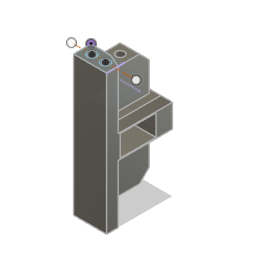
hinge_hood_front_v3 (Autodesk Fusion 360 design; units mm, degrees)
Autodesk Fusion 360 part; units mm, degrees
note: some values were not read from the file. Set by a fixed rule: which sketch regions a step uses.
sketch "Esquisse1" plane through (0, 0, 0) normal (0, 0, 1) x (1, 0, 0)
  line L0 (17, 0) -> (0, 0)
  line L1 (0, 0) -> (0, 72)
  line L2 (0, 72) -> (17, 72)
  line L3 (17, 72) -> (17, 0)
  dimension "d3" = 72
  dimension "d4" = 17
  constraint coincident L0.end L1.start
  constraint horizontal L0
  constraint perpendicular L0 L1
  constraint perpendicular L1 L2
  constraint perpendicular L0 L3
  measures "d3" distance of L0.end L1.end
  measures "d4" distance of L0.start L0.end
extrude "Extrusion1" add sketch "Esquisse1" along normal blind 9
sketch "Esquisse2" plane through (0, 0, 0) normal (0, -1, 0) x (1, 0, 0)
  line L0 (0, 0) -> (17, 0)
  line L1 (17, 9) -> (0, 9)
  line L2 (0, 9) -> (0, 0)
  line L3 (-5.7525, 4.5) -> (21.5406, 4.5) construction
  circle A0 centre (5, 4.5) radius 2.175
  circle A1 centre (12, 4.5) radius 2.175
  line L4 (17, 0) -> (17, 9)
  dimension "d7" = 4.35
  dimension "d8" = 7
  dimension "d9" = 4.5
  dimension "d10" = 5
  constraint coincident L3 A0.centre
  constraint coincident L3 A1.centre
  constraint equal A0 A1
  measures "d7" diameter of A0
  measures "d8" distance of A0.centre A1.centre
  measures "d9" vertical distance of L0.start L3.start
  measures "d10" distance of L2 A0.centre
extrude "Extrusion2" cut sketch "Esquisse2" against normal blind 8 contours A0 | A1
sketch "Esquisse3" plane through (0, 72, 0) normal (0, 1, 0) x (-1, 0, 0)
  line L0 (-17, 0) -> (0, 0)
  line L1 (0, 0) -> (0, 9)
  line L2 (0, 9) -> (-17, 9)
  line L3 (5.6122, 4.5) -> (-27.7174, 4.5) construction
  circle A0 centre (-12, 4.5) radius 2.175
  circle A1 centre (-5, 4.5) radius 2.175
  line L4 (-17, 9) -> (-17, 0)
  dimension "d13" = 4.5
  dimension "d14" = 7
  dimension "d15" = 5
  dimension "d16" = 4.35
  constraint coincident L3 A0.centre
  constraint coincident L3 A1.centre
  constraint equal A0 A1
  measures "d13" distance of L0.end L3
  measures "d14" distance of A0.centre A1.centre
  measures "d15" distance of L1 A1.centre
  measures "d16" diameter of A0
extrude "Extrusion3" cut sketch "Esquisse3" against normal blind 8 contours A0 | A1
sketch "Esquisse9" plane through (0, 0, 0) normal (-1, 0, 0) x (0, 0, 1)
  line L0 (0, 72) -> (0, 0)
  line L1 (0, 0) -> (9, 0)
  line L2 (9, 0) -> (9, 72)
  line L3 (9, 72) -> (0, 72)
  line L4 (9, 65) -> (-15, 65)
  line L5 (-15, 65) -> (-15, 48.5)
  line L6 (-15, 48.5) -> (9, 48.5)
  line L7 (9, 48.5) -> (9, 65)
  line L8 (9, 7) -> (-15, 7)
  line L9 (-15, 7) -> (-15, 23.5)
  line L10 (-15, 23.5) -> (9, 23.5)
  line L11 (9, 23.5) -> (9, 7)
  line L12 (6.675, 72) -> (2.325, 72)
  dimension "d48" = 7
  dimension "d49" = 7
  dimension "d50" = 25
  dimension "d51" = 15
  constraint horizontal L4
  constraint vertical L5
  constraint horizontal L6
  constraint vertical L7
  constraint coincident L2 L4.start
  constraint horizontal L8
  constraint vertical L9
  constraint horizontal L10
  constraint vertical L11
  constraint coincident L2 L8.start
  constraint equal L5 L9
  constraint collinear L5 L9
  measures "d48" distance of L1 L8
  measures "d49" distance of L4 L12
  measures "d50" distance of L6 L10
  measures "d51" distance of L0 L9
extrude "Extrusion7" add sketch "Esquisse9" against normal blind 10 contours L0 L4 L5 L6 | L0 L8 L9 L10
sketch "Esquisse10" plane through (0, 7, 0) normal (0, -1, 0) x (1, 0, 0)
  line L0 (0, -15) -> (10, -15)
  line L1 (10, -15) -> (10, 0)
  line L2 (10, 0) -> (0, 0)
  line L3 (0, 0) -> (0, -15)
  circle A0 centre (5, -10) radius 2.175
  dimension "d56" = 4.35
  dimension "d57" = 5
  dimension "d76" = 5
  measures "d56" diameter of A0
  measures "d57" distance of L0 A0.centre
  measures "d76" distance of L1 A0.centre
extrude "Extrusion9" cut sketch "Esquisse10" against normal blind 61 contours A0
sketch "Esquisse11" plane through (0, 48.5, 0) normal (0, -1, 0) x (1, 0, 0)
  circle A0 centre (5, -10) radius 2.175
  line L0 (10, -15) -> (10, 0)
  line L1 (10, 0) -> (0, 0)
  line L2 (0, 0) -> (0, -15)
  line L3 (0, -15) -> (10, -15)
chamfer "Chanfrein4" distance 7 distance2 3 1 edges at (17, 36, 0) measured on face at (3.3333, 40.1667, 0)
sketch "Esquisse12" plane through (0, 0, -15) normal (0, 0, -1) x (-1, 0, 0)
  line L0 (0, 48.5) -> (0, 65)
  line L1 (0, 65) -> (-10, 65)
  line L2 (-10, 65) -> (-10, 48.5)
  line L3 (-10, 48.5) -> (0, 48.5)
  line L4 (-10, 65) -> (0, 65)
  line L5 (0, 65) -> (0, 7)
  line L6 (0, 7) -> (-10, 7)
  line L7 (-10, 7) -> (-10, 65)
  line L8 (0, 7) -> (-10, 7)
  constraint horizontal L4
  constraint vertical L5
  constraint horizontal L6
  constraint vertical L7
  constraint coincident L1.end L2.start
  constraint collinear L6 L8
extrude "Extrusion10" add sketch "Esquisse12" along normal blind 10
extrude "Extrusion11" add 1 faces at (6.6667, 31.8333, -15) along direction (0, 0, 1) up to surface (15 mm away)
sketch "Esquisse13" plane through (0, 0, -25) normal (0, 0, -1) x (-1, 0, 0)
  line L0 (0, 7) -> (0, 65)
  line L1 (-10, 65) -> (-10, 7)
  line L2 (-10, 27) -> (-17, 27)
  line L3 (-17, 27) -> (-17, 45)
  line L4 (-17, 45) -> (-10, 45)
  line L5 (-10, 45) -> (-10, 27)
  line L6 (0, 65) -> (-10, 65)
  line L7 (-10, 7) -> (0, 7)
  dimension "d82" = 7
  constraint horizontal L2
  constraint vertical L3
  constraint horizontal L4
  constraint vertical L5
  constraint coincident L1 L2.start
  measures "d82" distance of L2.start L2.end
extrude "Extrusion12" add sketch "Esquisse13" against normal blind 28 contours L1 L2 L3 L4 L5
sketch "Esquisse15" plane through (17, 0, 0) normal (1, 0, 0) x (0, 0, -1)
  line L0 (-3, 45) -> (-3, 72)
  line L1 (-3, 72) -> (-9, 72)
  line L2 (-9, 72) -> (-9, 0)
  line L3 (-9, 0) -> (-3, 0)
  line L4 (16.5, 30.5) -> (-2, 30.5)
  line L5 (-2, 30.5) -> (-2, 41.5)
  line L6 (-2, 41.5) -> (16.5, 41.5)
  line L7 (16.5, 41.5) -> (16.5, 30.5)
  line L8 (-3, 0) -> (-3, 27)
  line L9 (-3, 27) -> (25, 27)
  line L10 (25, 27) -> (25, 45)
  line L11 (25, 45) -> (-3, 45)
  dimension "d96" = 7
  constraint horizontal L4
  constraint vertical L5
  constraint horizontal L6
  constraint vertical L7
  measures "d96" distance of L2 L5
extrude "Extrusion13" cut sketch "Esquisse15" against normal blind 27 contours L4 L5 L6 L7
chamfer "Chanfrein6" distance 3 angle 45 6 edges at (17, 27, -11) (17, 45, -11) (13.5, 27, -25) (13.5, 45, -25) (0, 41.5, -7.25) (0, 30.5, -7.25)
chamfer "Chanfrein7" distance 5 distance2 5 2 edges at (10, 53.5, -25) (10, 18.5, -25) measured on face at (3.3333, 34, -25) measured on face at (3.3333, 34, -25)
chamfer "Chanfrein8" distance 10 distance2 10 2 edges at (2.5, 65, -25) (2.5, 7, -25) measured on face at (13, 38, -25) measured on face at (13, 38, -25)
equation "d49 = d48"
